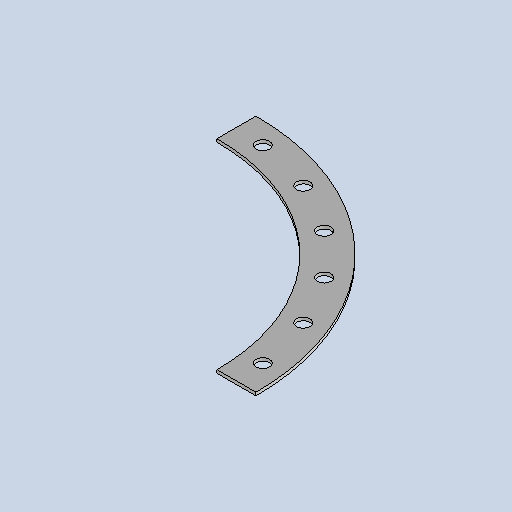
# Autodesk Inventor part: MSC 403 flange 500
Saved by Autodesk Inventor 2025 (Build 290162010, 162A)
## iProperties
Created: 2024-06-25
Part Number: MSC 403 flange 500
Material: Stainless Steel
Document SubType Name: Sheet Metal
Designer: pokla
Density: 8 g/cm^3
Sheet Metal Rule: AISI304 4mm Die 32
Appearance: Default
Flat Pattern Width: 30 cm
Flat Pattern Length: 30 cm
Flat Pattern Area: 900 cm^2
Sheet Metal Width: 300,000 mm
Sheet Metal Length: 300,000 mm
Sheet Metal Area: 90000,000 mm^2
Stock Number: МОО 403 фланец 500
Author: pokla
Autodesk Inventor part; units mm, degrees
ref_plane "YZ Plane" through (0, 0, 0) normal (1, 0, 0) x (0, 1, 0)
ref_plane "XZ Plane" through (0, 0, 0) normal (0, 1, 0) x (-1, 0, 0)
ref_plane "XY Plane" through (0, 0, 0) normal (0, 0, 1) x (1, 0, 0)
sketch "Sketch1" plane through (0, 0, 0) normal (0, 0, 1) x (1, 0, 0)
  arc A0 (251, 0) -> (0, 251) centre (0, 0) ccw
  arc A1 (0, 300) -> (300, 0) centre (0, 0) ccw construction
  circle A2 centre (0, 0) radius 320 construction
  line L0 (0, 0) -> (0, 251) construction
  line L1 (0, 0) -> (251, 0) construction
  arc A3 (300, 0) -> (0, 300) centre (0, 0) ccw
  line L2 (0, 251) -> (0, 300)
  arc A4 (0, 251) -> (251, 0) centre (0, 0) ccw construction
  line L3 (251, 0) -> (300, 0)
  dimension "d0" = 502
  dimension "d1" = 600
  dimension "d2" = 640
  measures "d0" diameter of A0
  measures "d1" diameter of A1
  measures "d2" diameter of A2
extrude "Plate1" add sketch "Sketch1" against normal blind 4
sketch "Sketch3" plane through (0, 0, 0) normal (0, 0, 1) x (1, 0, 0)
  circle A0 centre (0, 0) radius 275 construction
  line L0 (0, 0) -> (0, 300) construction
  arc A1 (300, 0) -> (0, 300) centre (0, 0) ccw projected
  line L1 (0, 0) -> (39.1579, 297.4335) construction
  circle A2 centre (35.8947, 272.6473) radius 8.5
  dimension "d12" = 550
  dimension "d13" = 7.5
  dimension "d14" = 17
  constraints: 4 end point, 2 point on circle, 1 centre point, 1 coincident, 1 point on line, 3 other
  measures "d13" angle of L0 L1
  measures "d14" diameter of A2
extrude "Extrusion2" cut sketch "Sketch3" against normal through all
pattern_circular "Circular Pattern1" count 6 over 75 about axis through (0, 0, -10) along (0, 0, -1) of "Extrusion2"
equation "\"d5\" = Thickness"
equation "\"BendReliefWidth\" = Thickness"
equation "\"BendReliefDepth\" = 0.5 * Thickness"
equation "\"CornerReliefSize\" = 4 * Thickness"
equation "\"MinimumRemnant\" = 2 * Thickness"
equation "\"TransitionRadius\" = BendRadius"
equation "\"JacobiRadiusSize\" = BendRadius"
equation "\"GapSize\" = Thickness"
equation "\"Thickness\" = 4"
equation "\"BendRadius\" = 6"
body "Solid1"
